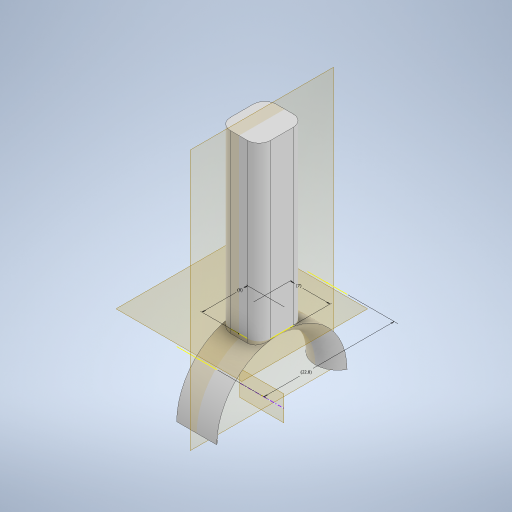
# Autodesk Inventor part: 막대2
Saved by Autodesk Inventor 2023 (Build 270158000, 158)
## iProperties
Created: 2023-04-26
Part Number: 막대2
Material: 일반
Document SubType Name: Modeling
Designer: rlatk
Density: 1 g/cm^3
Appearance: 기본값
Author: rlatk
Autodesk Inventor part; units mm, degrees
ref_plane "XZ Plane" through (0, 0, 0) normal (0, 1, 0) x (-1, 0, 0)
sketch "스케치1" plane through (0, 0, 0) normal (0, 1, 0) x (-1, 0, 0)
  line L0 (0, 0) -> (3.5, 0)
  line L1 (0, 0) -> (-3.5, 0)
  line L2 (3.5, 0) -> (-3.5, 0)
  arc A0 (3.5, 0) -> (-3.5, 0) centre (0, -1.9365) ccw
  dimension "d0" = 3.5
  dimension "d1" = 3.5
  dimension "d2" = 4
  constraints: 6 end point, 2 horizontal, 2 point on circle, 1 centre point, 1 collinear
  measures "d0" distance of L0.start L0.end
  measures "d1" distance of L0.start L1.end
  measures "d2" radius of A0
ref_plane "작업 평면1" through (0, 0, 11.4) normal (0, 0, 1) x (1, 0, 0)
sketch "스케치2" plane through (0, 0, 11.4) normal (0, 0, 1) x (1, 0, 0)
  line L0 (-3.8254, 0) -> (3.8254, 0)
  point P0 (0, 0)
  constraints: 2 end point, 1 horizontal
revolve "회전1" add sketch "스케치1" angle 180 about axis through (-3.8254, 0, 11.4) along (1, 0, 0)
ref_plane "작업 평면2" through (-3.5, 11.4, 11.4) normal (0, 1, 0) x (-1, 0, 0)
sketch "스케치3" plane through (-3.5, 11.4, 11.4) normal (0, 1, 0) x (-1, 0, 0)
  line L0 (0, 11.4) -> (0, -11.4) projected
  line L1 (-7, 11.4) -> (-7, -11.4) projected
  line L2 (0, 4) -> (-7, 4)
  line L3 (-7, 4) -> (-7, -4)
  line L4 (-7, -4) -> (0, -4)
  line L5 (0, -4) -> (0, 4)
  line L6 (-8.8556, 0) -> (1.8556, 0) projected
  point P0 (-3.5, -11.4)
  point P1 (-3.5, 4)
  point P2 (0, -4)
  point P3 (-7, 4)
  dimension "d5" = 4
  dimension "d6" = 4
  constraints: 8 end point, 2 parallel, 2 point on line, 1 horizontal, 1 midpoint, 1 perpendicular
  measures "d5" distance from line of point (-3.5, 4) L6
  measures "d6" distance between parallel lines of L4 L6
extrude "돌출1" add sketch "스케치3" along normal blind 30
sketch "스케치4" plane through (0, 0, 0) normal (1, 0, 0) x (0, 1, 0)
  line L0 (11.4, 15.4) -> (11.4, 11.4) projected
  line L1 (11.4, 15.4) -> (41.4, 15.4) projected
  line L2 (11.4, 11.4) -> (11.4, 15.4)
  line L3 (11.4, 15.4) -> (10.6752, 15.4)
  arc A0 (11.4, 11.4) -> (0, 22.8) centre (0, 11.4) ccw projected
  arc A1 (11.4, 11.4) -> (10.6752, 15.4) centre (0, 11.4) ccw
  line L4 (11.4, 11.4) -> (11.4, 7.4) projected
  line L5 (11.4, 11.4) -> (11.4, 7.4)
  line L6 (11.4, 7.4) -> (10.6752, 7.4)
  arc A2 (0, 0) -> (11.4, 11.4) centre (0, 11.4) ccw projected
  arc A3 (10.6752, 7.4) -> (11.4, 11.4) centre (0, 11.4) ccw
  constraints: 8 end point, 6 point on circle, 3 perpendicular, 2 centre point, 2 concentric, 1 collinear, 1 tangent
extrude "돌출2" add sketch "스케치4" along normal blind 3.5 and the other way blind 3.5
sketch "스케치5" plane through (-3.5, 11.4, 11.4) normal (0, 1, 0) x (-1, 0, 0)
  line L0 (-7, -4) -> (0, -4) projected
  line L1 (-7, 4) -> (-7, -4) projected
  line L2 (0, 4) -> (-7, 4) projected
  line L3 (0, -4) -> (0, 4) projected
  line L4 (-7, -4) -> (0, -4)
  line L5 (0, -4) -> (0, 4)
  line L6 (0, 4) -> (-7, 4)
  line L7 (-7, 4) -> (-7, -4)
  line L8 (-2.5, -2.5) -> (-4.5, -2.5)
  line L9 (-5.5, -1.5) -> (-5.5, 1.5)
  line L10 (-4.5, 2.5) -> (-2.5, 2.5)
  line L11 (-1.5, 1.5) -> (-1.5, -1.5)
  arc A0 (-2.5, -2.5) -> (-1.5, -1.5) centre (-2.5, -1.5) ccw
  arc A1 (-1.5, 1.5) -> (-2.5, 2.5) centre (-2.5, 1.5) ccw
  arc A2 (-4.5, 2.5) -> (-5.5, 1.5) centre (-4.5, 1.5) ccw
  arc A3 (-5.5, -1.5) -> (-4.5, -2.5) centre (-4.5, -1.5) ccw
  point P0 (-3.5, -11.4)
  point P1 (-1.5, -2.5)
  point P2 (-5.5, -2.5)
  point P3 (-5.5, 2.5)
  point P4 (-1.5, 2.5)
  dimension "d13" = 1.5
  dimension "d24" = 1
  constraints: 16 end point, 8 point on circle, 8 point on line, 8 tangent, 4 centre point, 3 equal radius, 2 parallel, 1 horizontal, 1 perpendicular, 3 other
  measures "d13" distance between parallel lines of L0 L8
  measures "d24" radius of A0
extrude "돌출3" cut sketch "스케치5" along normal blind 28 and the other way blind 5 contours L8 A3 L9 A2 L10 A1 L11 A0
sketch "스케치6" plane through (3.5, 41.4, 7.4) normal (0, 0, -1) x (-1, 0, 0)
  line L0 (5.5, -31.8494) -> (5.5, -2) projected
  line L1 (2.5, -2) -> (4.5, -2) projected
  line L2 (1.5, -31.8494) -> (1.5, -2) projected
  line L3 (4.5, -2) -> (2.5, -2)
  line L4 (1.5, -3) -> (1.5, -5)
  line L5 (2.5, -6) -> (4.5, -6)
  line L6 (5.5, -5) -> (5.5, -3)
  arc A0 (4.5, -6) -> (5.5, -5) centre (4.5, -5) ccw
  arc A1 (5.5, -3) -> (4.5, -2) centre (4.5, -3) ccw
  arc A2 (2.5, -2) -> (1.5, -3) centre (2.5, -3) ccw
  arc A3 (1.5, -5) -> (2.5, -6) centre (2.5, -5) ccw
  point P0 (3.5, -41.4)
  point P1 (1.5, -6)
  point P2 (1.5, -2)
  point P3 (5.5, -6)
  point P4 (1.5, -6)
  point P5 (5.5, -6)
  point P6 (1.5, -3)
  point P7 (2.5, -2)
  point P8 (5.5, -3)
  point P9 (5.5, -5)
  point P10 (1.5, -5)
  dimension "d18" = 4
  dimension "d19" = 4
  dimension "d23" = 1
  constraints: 8 end point, 8 point on circle, 8 point on line, 8 tangent, 4 centre point, 3 equal radius, 2 parallel, 1 horizontal, 1 perpendicular
  measures "d18" distance of point (5.5, -6) point (1.5, -6)
  measures "d19" distance of point (1.5, -6) point (1.5, -2)
  measures "d23" radius of A0
fillet "모깎기1" radius 2 4 edges at (-3.5, 26.0376, 7.4) (3.5, 26.0376, 7.4) (3.5, 26.0376, 15.4) (-3.5, 26.0376, 15.4)
extrude "돌출5" cut sketch "스케치6" against normal blind 3
sketch "스케치7" plane through (-3.5, 11.4, 11.4) normal (0, 1, 0) x (-1, 0, 0)
  line L0 (-7, 11.4) -> (0, 11.4) projected
  line L1 (-7, -11.4) -> (0, -11.4) projected
  line L2 (-2, 4) -> (-5, 4) projected
  line L3 (-5, -4) -> (-2, -4) projected
  line L4 (0, -2) -> (0, 2) projected
  line L5 (-7, 2) -> (-7, -2) projected
  point P0 (-3.5, -11.4)
  point P1 (-3.5, 4)
  point P2 (-3.5, -4)
  dimension "d27" = 22.8
  dimension "d28" = 8
  dimension "d29" = 7
  constraints: 2 midpoint
  measures "d27" distance between parallel lines of L0 L1
  measures "d28" distance of point (-3.5, 4) point (-3.5, -4)
  measures "d29" distance between parallel lines of L4 L5
